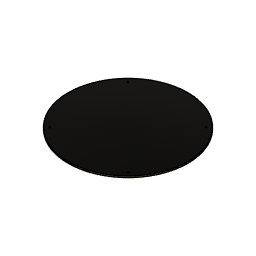
digitalclock_backside v3 (Autodesk Fusion 360 design; units mm, degrees)
Autodesk Fusion 360 part; units mm, degrees
sketch "Skizze1" plane through (0, 0, 0) normal (0, 0, 1) x (1, 0, 0)
  circle A0 centre (0, 0) radius 130
  dimension "d1" = 260
  constraint coincident A0.centre origin
  measures "d1" diameter of A0
extrude "Extrusion1" add sketch "Skizze1" along normal blind 3
sketch "Skizze3" plane through (0, 0, 0) normal (0, 0, -1) x (1, 0, 0)
  circle A0 centre (0, 0) radius 130
  circle A1 centre (-85, 85) radius 1.5
  circle A2 centre (-85, -85) radius 1.5
  circle A3 centre (85, -85) radius 1.5
  circle A4 centre (85, 85) radius 1.5
  dimension "d4" = 3
  dimension "d5" = 85
  dimension "d6" = 85
  dimension "d8" = 360
  measures "d4" diameter of A1
  measures "d5" horizontal distance of A0.centre A1.centre
  measures "d6" vertical distance of A0.centre A1.centre
extrude "Extrusion2" cut sketch "Skizze3" against normal blind 3 contours A1 | A2 | A3 | A4
chamfer "Fase1" distance 1.5 angle 45 4 edges at (-86.3985, -85.5424, 0) (83.6015, -85.5424, 0) (-86.3985, 84.4576, 0) (83.6015, 84.4576, 0)
